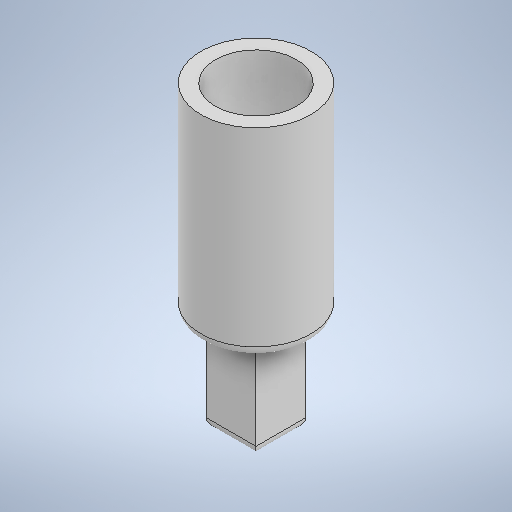
# Autodesk Inventor part: nut a
Saved by Autodesk Inventor 2025.1 (Build 291241020, 241B)
## iProperties
Created: 2025-01-27
Part Number: nut a
Material: Generic
Document SubType Name: Modeling
Designer: User
Density: 1 g/cm^3
Appearance: Default
Author: User
Autodesk Inventor part; units mm, degrees
ref_plane "YZ Plane" through (0, 0, 0) normal (1, 0, 0) x (0, 1, 0)
ref_plane "XZ Plane" through (0, 0, 0) normal (0, 1, 0) x (-1, 0, 0)
ref_plane "XY Plane" through (0, 0, 0) normal (0, 0, 1) x (1, 0, 0)
sketch "Sketch1" plane through (0, 0, 0) normal (0, 1, 0) x (-1, 0, 0)
  circle A0 centre (0, 0) radius 5.5
  line L0 (2.5, 2.5) -> (-2.5, 2.5)
  line L1 (-2.5, 2.5) -> (-2.5, -2.5)
  line L2 (-2.5, -2.5) -> (2.5, -2.5)
  line L3 (2.5, -2.5) -> (2.5, 2.5)
  line L4 (2.5, 2.5) -> (-2.5, -2.5) construction
  line L5 (-2.5, 2.5) -> (2.5, -2.5) construction
  dimension "d0" = 11
  dimension "d3" = 5
  dimension "d4" = 5
  constraints: 12 end point, 2 midpoint, 2 parallel, 1 centre point, 1 coincident, 1 horizontal, 1 perpendicular
  measures "d0" diameter of A0
  measures "d3" distance of L2.end L1.end
  measures "d4" distance of L0.end L1.end
extrude "Extrusion1" add sketch "Sketch1" along normal blind 10 contours A0 | L3 L2 L1 L0
extrude "Extrusion2" add sketch "Sketch1" against normal blind 10 contours L3 L2 L1 L0
fillet "Fillet1" radius 1 4 edges at (0, -10, -2.5) (-2.5, -10, 0) (0, -10, 2.5) (2.5, -10, 0)
fillet "Fillet2" radius 1 1 edges at (5.5, 0, 0)
sketch "Sketch2" plane through (0, 10, 0) normal (0, 1, 0) x (1, 0, 0)
  circle A0 centre (0, 0) radius 4.05
  circle A1 centre (0, 0) radius 5.5
  dimension "d9" = 8.1
  dimension "d10" = 11
  constraints: 2 centre point, 2 coincident
  measures "d9" diameter of A0
  measures "d10" diameter of A1
extrude "Extrusion3" cut sketch "Sketch2" against normal blind 5 contours A0
sketch "Sketch3" plane through (0, 10, 0) normal (0, 1, 0) x (1, 0, 0)
  point P0 (0, 0)
sketch "Sketch4" plane through (0, 10, 0) normal (0, 1, 0) x (1, 0, 0)
  circle A0 centre (0, 0) radius 5.5
  circle A1 centre (0, 0) radius 4.05
  dimension "d13" = 11
  constraints: 2 centre point, 2 coincident
  measures "d13" diameter of A0
extrude "Extrusion4" add sketch "Sketch4" along normal blind 10
body "Solid1"
